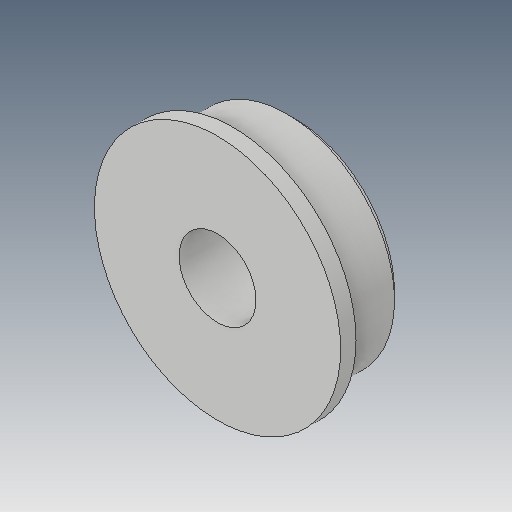
# Autodesk Inventor part: Flanged Bearing
Saved by Autodesk Inventor 2017 (Build 210142000, 142)
## iProperties
Created: 2016-07-20
Part Number: Flanged Bearing
Material: Generic
Document SubType Name: Modeling
Designer: User
Density: 1 g/cm^3
Appearance: Default
Mass: 0.713272 g
Surface Area: 6.54381 cm^2
Volume: 0.713272 cm^3
Author: User
Autodesk Inventor part; units mm, degrees
ref_plane "YZ Plane" through (0, 0, 0) normal (1, 0, 0) x (0, 1, 0)
ref_plane "XZ Plane" through (0, 0, 0) normal (0, 1, 0) x (-1, 0, 0)
ref_plane "XY Plane" through (0, 0, 0) normal (0, 0, 1) x (1, 0, 0)
sketch "Sketch1" plane through (0, 0, 0) normal (0, 0, 1) x (1, 0, 0)
  circle A0 centre (0, 0) radius 5.0674 projected
  circle A1 centre (0, 0) radius 2.5
  circle A2 centre (0, 0) radius 7
  point P0 (0, 0)
  dimension "d0" = 5
  dimension "d1" = 14
  constraints: 2 centre point, 2 coincident
  measures "d0" diameter of A1
  measures "d1" diameter of A2
extrude "Extrusion1" add sketch "Sketch1" along normal blind 5 contours A0 | A2
sketch "Sketch2" plane through (0, 0, 5) normal (0, 0, 1) x (1, 0, 0)
  circle A0 centre (0, 0) radius 2.5931
  circle A1 centre (0, 0) radius 2.5 projected
  circle A2 centre (0, 0) radius 8
  dimension "d4" = 16
  constraints: 2 centre point, 2 coincident
  measures "d4" diameter of A2
extrude "Extrusion2" add sketch "Sketch2" against normal blind 1 contours A2
chamfer "Chamfer1" distance 0.5 angle 45 1 edges at (-7, 0, 0)
body "Solid1"
